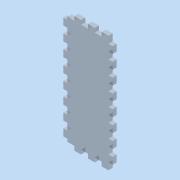
# Autodesk Inventor part: Bask_Wall
Saved by Autodesk Inventor 2015 (Build 190159000, 159)
## iProperties
Created: 2015-01-31
Part Number: Bask_Wall
Material: Wood (Birch)
Document SubType Name: Modeling
Designer: Openlab
Density: 0.55 g/cm^3
Appearance: Polycarbonate - Clear
Author: Openlab
Autodesk Inventor part; units mm, degrees
ref_plane "YZ Plane" through (0, 0, 0) normal (1, 0, 0) x (0, 1, 0)
ref_plane "XZ Plane" through (0, 0, 0) normal (0, 1, 0) x (-1, 0, 0)
ref_plane "XY Plane" through (0, 0, 0) normal (0, 0, 1) x (1, 0, 0)
sketch "Sketch1" plane through (0, 0, 0) normal (0, 1, 0) x (-1, 0, 0)
  line L0 (30, -5) -> (33, -5)
  line L1 (33, -5) -> (33, -10)
  line L2 (33, -10) -> (30, -10)
  line L3 (30, -15) -> (33, -15)
  line L4 (33, -15) -> (33, -20)
  line L5 (33, -20) -> (30, -20)
  line L6 (30, -25) -> (33, -25)
  line L7 (33, -25) -> (33, -30)
  line L8 (33, -30) -> (30, -30)
  line L9 (30, -35) -> (33, -35)
  line L10 (33, -35) -> (33, -40)
  line L11 (33, -40) -> (30, -40)
  line L12 (30, -45) -> (33, -45)
  line L13 (33, -45) -> (33, -50)
  line L14 (33, -50) -> (30, -50)
  line L15 (30, -55) -> (33, -55)
  line L16 (33, -55) -> (33, -60)
  line L17 (33, -60) -> (30, -60)
  line L18 (30, -65) -> (33, -65)
  line L19 (33, -65) -> (33, -70)
  line L20 (33, -70) -> (30, -70)
  line L21 (30, -75) -> (33, -75)
  line L22 (33, -75) -> (33, -80)
  line L23 (33, -80) -> (30, -80)
  line L24 (0, -5) -> (-3, -5)
  line L25 (-3, -5) -> (-3, -10)
  line L26 (-3, -10) -> (0, -10)
  line L27 (0, -15) -> (-3, -15)
  line L28 (-3, -20) -> (0, -20)
  line L29 (-3, -15) -> (-3, -20)
  line L30 (0, -25) -> (-3, -25)
  line L31 (-3, -25) -> (-3, -30)
  line L32 (-3, -30) -> (0, -30)
  line L33 (0, -35) -> (-3, -35)
  line L34 (-3, -35) -> (-3, -40)
  line L35 (-3, -40) -> (0, -40)
  line L36 (0, -45) -> (-3, -45)
  line L37 (-3, -45) -> (-3, -50)
  line L38 (-3, -50) -> (0, -50)
  line L39 (0, -55) -> (-3, -55)
  line L40 (-3, -55) -> (-3, -60)
  line L41 (-3, -60) -> (0, -60)
  line L42 (0, -65) -> (-3, -65)
  line L43 (-3, -65) -> (-3, -70)
  line L44 (-3, -70) -> (0, -70)
  line L45 (0, -75) -> (-3, -75)
  line L46 (-3, -75) -> (-3, -80)
  line L47 (-3, -80) -> (0, -80)
  line L48 (30, -3) -> (30, -5)
  line L49 (30, -10) -> (30, -15)
  line L50 (30, -20) -> (30, -25)
  line L51 (30, -30) -> (30, -35)
  line L52 (30, -40) -> (30, -45)
  line L53 (30, -50) -> (30, -55)
  line L54 (30, -60) -> (30, -65)
  line L55 (30, -70) -> (30, -75)
  line L56 (30, -80) -> (30, -82)
  line L57 (0, -5) -> (0, 0)
  line L58 (0, -15) -> (0, -10)
  line L59 (0, -25) -> (0, -20)
  line L60 (0, -35) -> (0, -30)
  line L61 (0, -45) -> (0, -40)
  line L62 (0, -55) -> (0, -50)
  line L63 (0, -65) -> (0, -60)
  line L64 (0, -85) -> (0, -80)
  line L65 (0, -75) -> (0, -70)
  line L66 (5, 0) -> (5, -3)
  line L67 (5, -3) -> (10, -3)
  line L68 (10, -3) -> (10, 0)
  line L69 (15, 0) -> (15, -3)
  line L70 (15, -3) -> (20, -3)
  line L71 (20, -3) -> (20, -0.0226)
  line L72 (25, -0.0226) -> (25, -3)
  line L73 (25, -3) -> (30, -3)
  line L74 (20, -0.0226) -> (25, -0.0226)
  line L75 (0, 0) -> (5, 0)
  line L76 (10, 0) -> (15, 0)
  line L77 (5, -85) -> (5, -82)
  line L78 (5, -82) -> (10, -82)
  line L79 (10, -82) -> (10, -85)
  line L80 (15, -85) -> (15, -82)
  line L81 (15, -82) -> (20, -82)
  line L82 (20, -82) -> (20, -85)
  line L83 (30, -82) -> (30, -82)
  line L84 (25, -85) -> (20, -85)
  line L85 (15, -85) -> (10, -85)
  line L86 (5, -85) -> (0, -85)
  line L87 (25, -85) -> (25, -82)
  line L88 (25, -82) -> (30, -82)
  constraints: 208 perpendicular, 178 end point, 99 parallel, 41 point on line, 5 horizontal, 2 vertical
extrude "Extrusion1" add sketch "Sketch1" along normal blind 3
body "Solid1"
